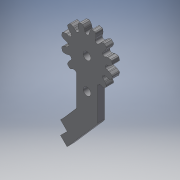
# Autodesk Inventor part: Part22
Saved by Autodesk Inventor 2019.2 (Build 232265000, 265)
## iProperties
Created: 2019-04-05
Part Number: Part22
Material: Generic
Document SubType Name: Modeling
Designer: richard.girt
Mass: 1.18335 g
Surface Area: 13.0931 cm^2
Volume: 1.18335 cm^3
Density: 1 g/cm^3
Appearance: Default
Author: richard.girt
Autodesk Inventor part; units mm, degrees
ref_plane "YZ Plane" through (0, 0, 0) normal (1, 0, 0) x (0, 1, 0)
ref_plane "XZ Plane" through (0, 0, 0) normal (0, 1, 0) x (-1, 0, 0)
ref_plane "XY Plane" through (0, 0, 0) normal (0, 0, 1) x (1, 0, 0)
sketch "Sketch1" plane through (0, 0, 0) normal (0, 0, 1) x (1, 0, 0)
  line L0 (-7.7681, -34.5191) -> (3.8225, -21.2975)
  arc A0 (3.8225, -21.2975) -> (4.0704, -20.6384) centre (3.0704, -20.6384) ccw
  line L1 (4.0704, -20.6384) -> (4.0704, -8.0614)
  line L2 (-4.0704, -8.0614) -> (-4.0704, -19.3318)
  arc A1 (-4.3183, -19.9909) -> (-4.0704, -19.3318) centre (-5.0704, -19.3318) ccw
  line L3 (-4.3183, -19.9909) -> (-9, -25.3753)
  line L4 (-9, -25.3753) -> (-10.3186, -26.694)
  line L5 (-10.3186, -26.694) -> (-7.6814, -29.3312)
  line L6 (-7.6814, -29.3312) -> (-10.3186, -31.9685)
  line L7 (-10.3186, -31.9685) -> (-7.7681, -34.5191)
  circle A2 centre (0, 0) radius 1.5
  arc A3 (-3.3755, 9.1889) -> (-3.4313, 8.1407) centre (0.2031, 8.473) ccw
  arc A4 (-3.0296, 9.6246) -> (-3.3755, 9.1889) centre (-2.8772, 9.1484) ccw
  arc A5 (-3.4313, 8.1407) -> (-3.3708, 7.8116) centre (-1.3483, 8.3535) ccw
  line L8 (-3.3708, 7.8116) -> (-3.1791, 7.0961)
  arc A6 (-3.5625, 6.1704) -> (-3.1791, 7.0961) centre (-3.974, 6.8831) ccw
  arc A7 (-1.1439, 8.86) -> (-1.6711, 9.6456) centre (-4.4124, 7.2363) ccw
  arc A8 (-1.6711, 9.6456) -> (-2.1886, 9.85) centre (-2.0825, 9.3614) ccw
  arc A9 (-0.9866, 8.4504) -> (-1.1439, 8.86) centre (-3.0091, 7.9085) ccw
  line L9 (-0.9866, 8.4504) -> (-0.7949, 7.7349)
  arc A10 (-0.7949, 7.7349) -> (0, 7.125) centre (0, 7.9479) ccw
  line L10 (-3.0296, 9.6246) -> (-2.1886, 9.85)
  arc A11 (-7.5177, 6.27) -> (-7.0419, 5.3344) centre (-4.0606, 7.4393) ccw
  arc A12 (-7.436, 6.8204) -> (-7.5177, 6.27) centre (-7.0659, 6.4842) ccw
  arc A13 (-7.101, 5.4207) -> (-6.825, 5.0796) centre (-5.3444, 6.5602) ccw
  line L11 (-6.825, 5.0796) -> (-6.3012, 4.5559)
  arc A14 (-6.1704, 3.5625) -> (-6.3012, 4.5559) centre (-6.8831, 3.974) ccw
  arc A15 (-5.4207, 7.101) -> (-6.27, 7.5177) centre (-7.4393, 4.0606) ccw
  arc A16 (-6.27, 7.5177) -> (-6.8204, 7.436) centre (-6.4842, 7.0659) ccw
  arc A17 (-5.0796, 6.825) -> (-5.4207, 7.101) centre (-6.5602, 5.3444) ccw
  line L12 (-5.0796, 6.825) -> (-4.5559, 6.3012)
  arc A18 (-4.5559, 6.3012) -> (-3.5625, 6.1704) centre (-3.974, 6.8831) ccw
  line L13 (-7.436, 6.8204) -> (-6.8204, 7.436)
  arc A19 (-9.6456, 1.6711) -> (-8.86, 1.1439) centre (-7.2363, 4.4124) ccw
  arc A20 (-9.85, 2.1886) -> (-9.6456, 1.6711) centre (-9.3614, 2.0825) ccw
  arc A21 (-8.86, 1.1439) -> (-8.4504, 0.9866) centre (-7.9085, 3.0091) ccw
  line L14 (-8.4504, 0.9866) -> (-7.7349, 0.7949)
  arc A22 (-7.125, 0) -> (-7.7349, 0.7949) centre (-7.9479, 0) ccw
  arc A23 (-8.1407, 3.4313) -> (-9.1889, 3.3755) centre (-8.473, -0.2031) ccw
  arc A24 (-9.1889, 3.3755) -> (-9.6246, 3.0296) centre (-9.1484, 2.8772) ccw
  arc A25 (-7.8116, 3.3708) -> (-8.2449, 3.4393) centre (-8.3535, 1.3483) ccw
  line L15 (-7.8116, 3.3708) -> (-7.0961, 3.1791)
  arc A26 (-7.0961, 3.1791) -> (-6.1704, 3.5625) centre (-6.8831, 3.974) ccw
  line L16 (-9.85, 2.1886) -> (-9.6246, 3.0296)
  arc A27 (-9.1889, -3.3755) -> (-8.2449, -3.4393) centre (-8.473, 0.2031) ccw
  arc A28 (-9.6246, -3.0296) -> (-9.1889, -3.3755) centre (-9.1484, -2.8772) ccw
  arc A29 (-8.2449, -3.4393) -> (-7.8116, -3.3708) centre (-8.3535, -1.3483) ccw
  line L17 (-7.8116, -3.3708) -> (-7.0961, -3.1791)
  arc A30 (-6.1704, -3.5625) -> (-7.0961, -3.1791) centre (-6.8831, -3.974) ccw
  arc A31 (-8.86, -1.1439) -> (-9.6456, -1.6711) centre (-7.2363, -4.4124) ccw
  arc A32 (-9.6456, -1.6711) -> (-9.85, -2.1886) centre (-9.3614, -2.0825) ccw
  arc A33 (-8.4504, -0.9866) -> (-8.86, -1.1439) centre (-7.9085, -3.0091) ccw
  line L18 (-8.4504, -0.9866) -> (-7.7349, -0.7949)
  arc A34 (-7.7349, -0.7949) -> (-7.125, 0) centre (-7.9479, 0) ccw
  line L19 (-9.6246, -3.0296) -> (-9.85, -2.1886)
  arc A35 (-6.27, -7.5177) -> (-5.5799, -7.2009) centre (-7.4393, -4.0606) ccw
  arc A36 (-4.0704, -8.0614) -> (-5.5799, -7.2009) centre (-5.0704, -8.0614) ccw
  arc A37 (-6.8204, -7.436) -> (-6.27, -7.5177) centre (-6.4842, -7.0659) ccw
  arc A38 (-7.101, -5.4207) -> (-7.5177, -6.27) centre (-4.0606, -7.4393) ccw
  arc A39 (-7.5177, -6.27) -> (-7.436, -6.8204) centre (-7.0659, -6.4842) ccw
  arc A40 (-6.825, -5.0796) -> (-7.101, -5.4207) centre (-5.3444, -6.5602) ccw
  line L20 (-6.825, -5.0796) -> (-6.3012, -4.5559)
  arc A41 (-6.3012, -4.5559) -> (-6.1704, -3.5625) centre (-6.8831, -3.974) ccw
  line L21 (-6.8204, -7.436) -> (-7.436, -6.8204)
  arc A42 (7.5177, -6.27) -> (7.0419, -5.3344) centre (4.0606, -7.4393) ccw
  arc A43 (7.436, -6.8204) -> (7.5177, -6.27) centre (7.0659, -6.4842) ccw
  arc A44 (7.0419, -5.3344) -> (6.825, -5.0796) centre (5.3444, -6.5602) ccw
  line L22 (6.825, -5.0796) -> (6.3012, -4.5559)
  arc A45 (6.1704, -3.5625) -> (6.3012, -4.5559) centre (6.8831, -3.974) ccw
  arc A46 (5.5799, -7.2009) -> (6.27, -7.5177) centre (7.4393, -4.0606) ccw
  arc A47 (5.5799, -7.2009) -> (4.0704, -8.0614) centre (5.0704, -8.0614) ccw
  arc A48 (6.27, -7.5177) -> (6.8204, -7.436) centre (6.4842, -7.0659) ccw
  line L23 (7.436, -6.8204) -> (6.8204, -7.436)
  arc A49 (9.6456, -1.6711) -> (8.7657, -1.0988) centre (7.2363, -4.4124) ccw
  arc A50 (9.85, -2.1886) -> (9.6456, -1.6711) centre (9.3614, -2.0825) ccw
  arc A51 (8.7657, -1.0988) -> (8.4504, -0.9866) centre (7.9085, -3.0091) ccw
  line L24 (8.4504, -0.9866) -> (7.7349, -0.7949)
  arc A52 (7.125, 0) -> (7.7349, -0.7949) centre (7.9479, 0) ccw
  arc A53 (8.1407, -3.4313) -> (9.1889, -3.3755) centre (8.473, 0.2031) ccw
  arc A54 (9.1889, -3.3755) -> (9.6246, -3.0296) centre (9.1484, -2.8772) ccw
  arc A55 (7.8116, -3.3708) -> (8.2449, -3.4393) centre (8.3535, -1.3483) ccw
  line L25 (7.8116, -3.3708) -> (7.0961, -3.1791)
  arc A56 (7.0961, -3.1791) -> (6.1704, -3.5625) centre (6.8831, -3.974) ccw
  line L26 (9.85, -2.1886) -> (9.6246, -3.0296)
  arc A57 (9.1889, 3.3755) -> (8.1407, 3.4313) centre (8.473, -0.2031) ccw
  arc A58 (9.6246, 3.0296) -> (9.1889, 3.3755) centre (9.1484, 2.8772) ccw
  arc A59 (8.1407, 3.4313) -> (7.8116, 3.3708) centre (8.3535, 1.3483) ccw
  line L27 (7.8116, 3.3708) -> (7.0961, 3.1791)
  arc A60 (6.1704, 3.5625) -> (7.0961, 3.1791) centre (6.8831, 3.974) ccw
  arc A61 (8.86, 1.1439) -> (9.6456, 1.6711) centre (7.2363, 4.4124) ccw
  arc A62 (9.6456, 1.6711) -> (9.85, 2.1886) centre (9.3614, 2.0825) ccw
  arc A63 (8.4504, 0.9866) -> (8.86, 1.1439) centre (7.9085, 3.0091) ccw
  line L28 (8.4504, 0.9866) -> (7.7349, 0.7949)
  arc A64 (7.7349, 0.7949) -> (7.125, 0) centre (7.9479, 0) ccw
  line L29 (9.6246, 3.0296) -> (9.85, 2.1886)
  arc A65 (6.27, 7.5177) -> (5.4207, 7.101) centre (7.4393, 4.0606) ccw
  arc A66 (6.8204, 7.436) -> (6.27, 7.5177) centre (6.4842, 7.0659) ccw
  arc A67 (5.4207, 7.101) -> (5.0796, 6.825) centre (6.5602, 5.3444) ccw
  line L30 (5.0796, 6.825) -> (4.5559, 6.3012)
  arc A68 (3.5625, 6.1704) -> (4.5559, 6.3012) centre (3.974, 6.8831) ccw
  arc A69 (7.0419, 5.3344) -> (7.5177, 6.27) centre (4.0606, 7.4393) ccw
  arc A70 (7.5177, 6.27) -> (7.436, 6.8204) centre (7.0659, 6.4842) ccw
  arc A71 (6.825, 5.0796) -> (7.0419, 5.3344) centre (5.3444, 6.5602) ccw
  line L31 (6.825, 5.0796) -> (6.3012, 4.5559)
  arc A72 (6.3012, 4.5559) -> (6.1704, 3.5625) centre (6.8831, 3.974) ccw
  line L32 (6.8204, 7.436) -> (7.436, 6.8204)
  arc A73 (1.6711, 9.6456) -> (1.1439, 8.86) centre (4.4124, 7.2363) ccw
  arc A74 (2.1886, 9.85) -> (1.6711, 9.6456) centre (2.0825, 9.3614) ccw
  arc A75 (1.1439, 8.86) -> (0.9866, 8.4504) centre (3.0091, 7.9085) ccw
  line L33 (0.9866, 8.4504) -> (0.7949, 7.7349)
  arc A76 (0, 7.125) -> (0.7949, 7.7349) centre (0, 7.9479) ccw
  arc A77 (3.4313, 8.1407) -> (3.3755, 9.1889) centre (-0.2031, 8.473) ccw
  arc A78 (3.3755, 9.1889) -> (3.0296, 9.6246) centre (2.8772, 9.1484) ccw
  arc A79 (3.3708, 7.8116) -> (3.4393, 8.2449) centre (1.3483, 8.3535) ccw
  line L34 (3.3708, 7.8116) -> (3.1791, 7.0961)
  arc A80 (3.1791, 7.0961) -> (3.5625, 6.1704) centre (3.974, 6.8831) ccw
  line L35 (2.1886, 9.85) -> (3.0296, 9.6246)
  dimension "d0" = 3
  constraints: 196 point on circle, 81 centre point, 72 end point
  measures "d0" diameter of A2
extrude "Extrusion1" add sketch "Sketch1" along normal mid plane 2.8
sketch "Sketch2" plane through (0, 0, 1.4) normal (0, 0, 1) x (1, 0, 0)
  circle A0 centre (0, 0) radius 1.5 construction
  circle A1 centre (0, -7) radius 1.5
  line L0 (0, 0) -> (0, -7)
  dimension "d3" = 3
  dimension "d4" = 7
  constraints: 2 end point, 1 centre point, 1 vertical
  measures "d3" diameter of A1
  measures "d4" distance of L0.start L0.end
extrude "Extrusion2" cut sketch "Sketch2" against normal through all
body "Solid1"
